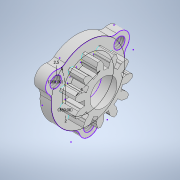
# Autodesk Inventor part: m1歯数11ギア6td6
Saved by Autodesk Inventor 2020.2 (Build 242310000, 310)
## iProperties
Created: 2020-02-29
Part Number: m1歯数11ギア6td6
Material: 一般
Document SubType Name: Modeling
Designer: aoyam
Density: 1 g/cm^3
Appearance: 既定
Author: aoyam
Autodesk Inventor part; units mm, degrees
ref_plane "YZ Plane" through (0, 0, 0) normal (1, 0, 0) x (0, 1, 0)
ref_plane "XZ Plane" through (0, 0, 0) normal (0, 1, 0) x (-1, 0, 0)
ref_plane "XY Plane" through (0, 0, 0) normal (0, 0, 1) x (1, 0, 0)
sketch "スケッチ1" plane through (0, 0, 0) normal (1, 0, 0) x (0, 1, 0)
  arc A0 (3.9405, 8.9701) -> (3.9064, 8.8492) centre (4.5356, 8.7369) ccw
  arc A1 (4.1405, 9.35) -> (3.9405, 8.9701) centre (5.6048, 8.3365) ccw
  arc A2 (4.786, 10.0383) -> (4.1405, 9.35) centre (6.7489, 7.5504) ccw
  arc A3 (2.588, 8.8492) -> (2.5538, 8.9701) centre (1.9587, 8.7369) ccw
  arc A4 (2.5538, 8.9701) -> (2.3538, 9.35) centre (0.8895, 8.3365) ccw
  arc A5 (2.3538, 9.35) -> (1.7083, 10.0383) centre (-0.2546, 7.5504) ccw
  arc A6 (3.7892, 7.9384) -> (2.7051, 7.9384) centre (3.2472, 3.7231) ccw
  arc A7 (1.7083, 10.0383) -> (1.1275, 9.8677) centre (3.2472, 3.7231) ccw
  line L0 (3.7892, 7.9384) -> (3.9064, 8.8492)
  line L1 (2.7051, 7.9384) -> (2.588, 8.8492)
  arc A8 (-0.1729, 7.7623) -> (-0.5466, 7.9738) centre (-1.2304, 6.3295) ccw
  arc A9 (-0.5466, 7.9738) -> (-1.4617, 8.2038) centre (-1.768, 5.0496) ccw
  arc A10 (-1.4617, 8.2038) -> (-1.8581, 7.7463) centre (3.2472, 3.7231) ccw
  arc A11 (0.9937, 8.512) -> (1.0303, 8.3918) centre (1.6204, 8.6376) ccw
  arc A12 (-0.0788, 7.679) -> (-0.1729, 7.7623) centre (-0.5474, 7.2444) ccw
  line L2 (0.5122, 6.9761) -> (-0.0788, 7.679)
  arc A13 (1.4242, 7.5623) -> (0.5122, 6.9761) centre (3.2472, 3.7231) ccw
  line L3 (1.4242, 7.5623) -> (1.0303, 8.3918)
  arc A14 (0.9565, 8.9398) -> (0.9937, 8.512) centre (2.7363, 8.8787) ccw
  arc A15 (1.1275, 9.8677) -> (0.9565, 8.9398) centre (4.1238, 8.836) ccw
  arc A16 (-1.8137, 5.2721) -> (-2.2424, 5.248) centre (-1.9287, 3.495) ccw
  arc A17 (-2.2424, 5.248) -> (-3.1366, 4.9467) centre (-1.689, 2.1277) ccw
  arc A18 (-3.1366, 4.9467) -> (-3.2228, 4.3475) centre (3.2472, 3.7231) ccw
  arc A19 (-1.2377, 6.5334) -> (-1.1419, 6.4522) centre (-0.7783, 6.9779) ccw
  arc A20 (-1.6895, 5.2529) -> (-1.8137, 5.2721) centre (-1.8488, 4.6339) ccw
  line L4 (-0.8124, 4.9811) -> (-1.6895, 5.2529)
  arc A21 (-0.362, 5.9672) -> (-0.8124, 4.9811) centre (3.2472, 3.7231) ccw
  line L5 (-0.362, 5.9672) -> (-1.1419, 6.4522)
  arc A22 (-1.5002, 6.8732) -> (-1.2377, 6.5334) centre (0.0301, 7.7841) ccw
  arc A23 (-1.8581, 7.7463) -> (-1.5002, 6.8732) centre (1.2204, 8.4983) ccw
  arc A24 (-1.8478, 2.2901) -> (-2.1954, 2.038) centre (-0.9838, 0.7329) ccw
  arc A25 (-2.1954, 2.038) -> (-2.7848, 1.3011) centre (-0.0429, -0.2878) ccw
  arc A26 (-2.7848, 1.3011) -> (-2.5333, 0.7505) centre (3.2472, 3.7231) ccw
  arc A27 (-2.0452, 3.6626) -> (-1.9206, 3.646) centre (-1.899, 4.2848) ccw
  arc A28 (-1.7329, 2.3411) -> (-1.8478, 2.2901) centre (-1.5323, 1.7342) ccw
  line L6 (-0.8481, 2.5866) -> (-1.7329, 2.3411)
  arc A29 (-1.0024, 3.6597) -> (-0.8481, 2.5866) centre (3.2472, 3.7231) ccw
  line L7 (-1.0024, 3.6597) -> (-1.9206, 3.646)
  arc A30 (-2.4497, 3.8065) -> (-2.0452, 3.6626) centre (-1.6548, 5.4002) ccw
  arc A31 (-3.2228, 4.3475) -> (-2.4497, 3.8065) centre (-1.0396, 6.6445) ccw
  arc A32 (-0.2643, -0.237) -> (-0.4204, -0.637) centre (1.3045, -1.0799) ccw
  arc A33 (-0.4204, -0.637) -> (-0.5178, -1.5755) centre (2.6478, -1.4298) ccw
  arc A34 (-0.5178, -1.5755) -> (-0.0086, -1.9028) centre (3.2472, 3.7231) ccw
  arc A35 (-1.1723, 0.811) -> (-1.0586, 0.8644) centre (-1.3858, 1.4134) ccw
  arc A36 (-0.1952, -0.132) -> (-0.2643, -0.237) centre (0.3017, -0.534) ccw
  line L8 (0.4164, 0.553) -> (-0.1952, -0.132)
  arc A37 (-0.2935, 1.3723) -> (0.4164, 0.553) centre (3.2472, 3.7231) ccw
  line L9 (-0.2935, 1.3723) -> (-1.0586, 0.8644)
  arc A38 (-1.5905, 0.7133) -> (-1.1723, 0.811) centre (-1.7833, 2.4837) ccw
  arc A39 (-2.5333, 0.7505) -> (-1.5905, 0.7133) centre (-1.9385, 3.8632) ccw
  arc A40 (2.4341, -1.5068) -> (2.519, -1.9277) centre (4.2096, -1.3677) ccw
  arc A41 (2.519, -1.9277) -> (2.9445, -2.7699) centre (5.5288, -0.9358) ccw
  arc A42 (2.9445, -2.7699) -> (3.5498, -2.7699) centre (3.2472, 3.7231) ccw
  arc A43 (1.1036, -1.1161) -> (1.1705, -1.0097) centre (0.5984, -0.7247) ccw
  arc A44 (2.4355, -1.3811) -> (2.4341, -1.5068) centre (3.0708, -1.4507) ccw
  line L10 (2.5797, -0.4742) -> (2.4355, -1.3811)
  arc A45 (1.5395, -0.1688) -> (2.5797, -0.4742) centre (3.2472, 3.7231) ccw
  line L11 (1.5395, -0.1688) -> (1.1705, -1.0097)
  arc A46 (0.8047, -1.4243) -> (1.1036, -1.1161) centre (-0.3147, -0.0392) ccw
  arc A47 (-0.0086, -1.9028) -> (0.8047, -1.4243) centre (-1.1911, 1.0373) ccw
  arc A48 (5.3907, -1.1161) -> (5.6896, -1.4243) centre (6.809, -0.0392) ccw
  arc A49 (5.6896, -1.4243) -> (6.5029, -1.9028) centre (7.6854, 1.0373) ccw
  arc A50 (6.5029, -1.9028) -> (7.0121, -1.5755) centre (3.2472, 3.7231) ccw
  arc A51 (4.0602, -1.5068) -> (4.0588, -1.3811) centre (3.4235, -1.4507) ccw
  arc A52 (5.3238, -1.0097) -> (5.3907, -1.1161) centre (5.896, -0.7247) ccw
  line L12 (4.9549, -0.1688) -> (5.3238, -1.0097)
  arc A53 (3.9146, -0.4742) -> (4.9549, -0.1688) centre (3.2472, 3.7231) ccw
  line L13 (3.9146, -0.4742) -> (4.0588, -1.3811)
  arc A54 (3.9753, -1.9277) -> (4.0602, -1.5068) centre (2.2848, -1.3677) ccw
  arc A55 (3.5498, -2.7699) -> (3.9753, -1.9277) centre (0.9655, -0.9358) ccw
  arc A56 (7.6666, 0.811) -> (8.0848, 0.7133) centre (8.2777, 2.4837) ccw
  arc A57 (8.0848, 0.7133) -> (9.0276, 0.7505) centre (8.4329, 3.8632) ccw
  arc A58 (9.0276, 0.7505) -> (9.2791, 1.3011) centre (3.2472, 3.7231) ccw
  arc A59 (6.7586, -0.237) -> (6.6895, -0.132) centre (6.1926, -0.534) ccw
  arc A60 (7.5529, 0.8644) -> (7.6666, 0.811) centre (7.8801, 1.4134) ccw
  line L14 (6.7878, 1.3723) -> (7.5529, 0.8644)
  arc A61 (6.0779, 0.553) -> (6.7878, 1.3723) centre (3.2472, 3.7231) ccw
  line L15 (6.0779, 0.553) -> (6.6895, -0.132)
  arc A62 (6.9147, -0.637) -> (6.7586, -0.237) centre (5.1898, -1.0799) ccw
  arc A63 (7.0121, -1.5755) -> (6.9147, -0.637) centre (3.8465, -1.4298) ccw
  arc A64 (8.5395, 3.6626) -> (8.944, 3.8065) centre (8.1491, 5.4002) ccw
  arc A65 (8.944, 3.8065) -> (9.7171, 4.3475) centre (7.5339, 6.6445) ccw
  arc A66 (9.7171, 4.3475) -> (9.6309, 4.9467) centre (3.2472, 3.7231) ccw
  arc A67 (8.3421, 2.2901) -> (8.2273, 2.3411) centre (8.0266, 1.7342) ccw
  arc A68 (8.4149, 3.646) -> (8.5395, 3.6626) centre (8.3933, 4.2848) ccw
  line L16 (7.4967, 3.6597) -> (8.4149, 3.646)
  arc A69 (7.3424, 2.5866) -> (7.4967, 3.6597) centre (3.2472, 3.7231) ccw
  line L17 (7.3424, 2.5866) -> (8.2273, 2.3411)
  arc A70 (8.6897, 2.038) -> (8.3421, 2.2901) centre (7.4781, 0.7329) ccw
  arc A71 (9.2791, 1.3011) -> (8.6897, 2.038) centre (6.5372, -0.2878) ccw
  arc A72 (7.732, 6.5334) -> (7.9945, 6.8732) centre (6.4643, 7.7841) ccw
  arc A73 (7.9945, 6.8732) -> (8.3524, 7.7463) centre (5.2739, 8.4983) ccw
  arc A74 (8.3524, 7.7463) -> (7.956, 8.2038) centre (3.2472, 3.7231) ccw
  arc A75 (8.3081, 5.2721) -> (8.1839, 5.2529) centre (8.3431, 4.6339) ccw
  arc A76 (7.6362, 6.4522) -> (7.732, 6.5334) centre (7.2727, 6.9779) ccw
  line L18 (6.8563, 5.9672) -> (7.6362, 6.4522)
  arc A77 (7.3067, 4.9811) -> (6.8563, 5.9672) centre (3.2472, 3.7231) ccw
  line L19 (7.3067, 4.9811) -> (8.1839, 5.2529)
  arc A78 (8.7367, 5.248) -> (8.3081, 5.2721) centre (8.4231, 3.495) ccw
  arc A79 (9.6309, 4.9467) -> (8.7367, 5.248) centre (8.1833, 2.1277) ccw
  arc A80 (5.5007, 8.512) -> (5.5378, 8.9398) centre (3.758, 8.8787) ccw
  arc A81 (5.5378, 8.9398) -> (5.3668, 9.8677) centre (2.3705, 8.836) ccw
  arc A82 (5.3668, 9.8677) -> (4.786, 10.0383) centre (3.2472, 3.7231) ccw
  arc A83 (6.6672, 7.7623) -> (6.5731, 7.679) centre (7.0417, 7.2444) ccw
  arc A84 (5.464, 8.3918) -> (5.5007, 8.512) centre (4.8739, 8.6376) ccw
  line L20 (5.0701, 7.5623) -> (5.464, 8.3918)
  arc A85 (5.9821, 6.9761) -> (5.0701, 7.5623) centre (3.2472, 3.7231) ccw
  line L21 (5.9821, 6.9761) -> (6.5731, 7.679)
  arc A86 (7.0409, 7.9738) -> (6.6672, 7.7623) centre (7.7247, 6.3295) ccw
  arc A87 (7.956, 8.2038) -> (7.0409, 7.9738) centre (8.2623, 5.0496) ccw
  circle A88 centre (3.2472, 3.7231) radius 3
  circle A89 centre (7.1594, 10.9864) radius 1.25
  arc A90 (9.3549, 10.4941) -> (5.5402, 12.5487) centre (7.1594, 10.9864) ccw
  arc A91 (9.3549, 10.4941) -> (9.7339, 8.8206) centre (11.3064, 10.0564) ccw
  arc A92 (3.9344, 11.9444) -> (5.5402, 12.5487) centre (4.101, 13.9374) ccw
  circle A93 centre (-4.9992, 3.4795) radius 1.25
  arc A94 (-5.6706, 5.627) -> (-4.4108, 6.792) centre (-6.2673, 7.5359) ccw
  arc A95 (-5.6706, 5.627) -> (-5.5426, 1.2961) centre (-4.9992, 3.4795) ccw
  arc A96 (-4.2163, 0.2076) -> (-5.5426, 1.2961) centre (-6.0257, -0.6447) ccw
  circle A97 centre (7.5813, -3.2967) radius 1.25
  arc A98 (6.0571, -4.9519) -> (4.4184, -4.4434) centre (4.7023, -6.4231) ccw
  arc A99 (6.0571, -4.9519) -> (9.7439, -2.6756) centre (7.5813, -3.2967) ccw
  arc A100 (10.0234, -0.9827) -> (9.7439, -2.6756) centre (11.6662, -2.1236) ccw
  arc A101 (10.0234, -0.9827) -> (9.7339, 8.8206) centre (3.2472, 3.7231) ccw
  arc A102 (3.9344, 11.9444) -> (-4.4108, 6.792) centre (3.2472, 3.7231) ccw
  arc A103 (-4.2163, 0.2076) -> (4.4184, -4.4434) centre (3.2472, 3.7231) ccw
  point P0 (0, 0)
  point P1 (5.4986, 8.5025)
  point P2 (5.538, 8.9335)
  point P3 (5.3668, 9.8677)
  point P4 (4.786, 10.0383)
  point P5 (4.137, 9.3449)
  point P6 (3.937, 8.9611)
  point P7 (3.9064, 8.8492)
  point P8 (3.7892, 7.9384)
  point P9 (2.7051, 7.9384)
  point P10 (2.5573, 8.9611)
  point P11 (2.3573, 9.3449)
  point P12 (1.7083, 10.0383)
  point P13 (1.1275, 9.8677)
  point P14 (0.9563, 8.9335)
  point P15 (0.9956, 8.5025)
  point P16 (1.4242, 7.5623)
  point P17 (0.5122, 6.9761)
  point P18 (-0.1651, 7.7565)
  point P19 (-0.5408, 7.9714)
  point P20 (-1.4617, 8.2038)
  point P21 (-1.8581, 7.7463)
  point P22 (-1.497, 6.8679)
  point P23 (-1.2309, 6.5265)
  point P24 (-1.1419, 6.4522)
  point P25 (-0.362, 5.9672)
  point P26 (-0.8124, 4.9811)
  point P27 (-1.8041, 5.2714)
  point P28 (-2.2363, 5.2491)
  point P29 (-3.1366, 4.9467)
  point P30 (-3.2228, 4.3475)
  point P31 (-2.4441, 3.8038)
  point P32 (-2.0357, 3.6605)
  point P33 (-1.9206, 3.646)
  point P34 (-1.0024, 3.6597)
  point P35 (-0.8481, 2.5866)
  point P36 (-1.8393, 2.2947)
  point P37 (-2.1908, 2.0422)
  point P38 (-2.7848, 1.3011)
  point P39 (-2.5333, 0.7505)
  point P40 (-1.5842, 0.714)
  point P41 (-1.1632, 0.8143)
  point P42 (-0.2597, -0.2285)
  point P43 (-0.4188, -0.6309)
  point P44 (-0.5178, -1.5755)
  point P45 (-0.0086, -1.9028)
  point P46 (0.8095, -1.4203)
  point P47 (1.1095, -1.1084)
  point P48 (2.5797, -0.4742)
  point P49 (2.4334, -1.4971)
  point P50 (2.5171, -1.9217)
  point P51 (2.9445, -2.7699)
  point P52 (3.5498, -2.7699)
  point P53 (3.9772, -1.9217)
  point P54 (4.061, -1.4971)
  point P55 (5.3848, -1.1084)
  point P56 (5.6848, -1.4203)
  point P57 (6.5029, -1.9028)
  point P58 (7.0121, -1.5755)
  point P59 (6.9131, -0.6309)
  point P60 (6.754, -0.2285)
  point P61 (6.6895, -0.132)
  point P62 (6.0779, 0.553)
  point P63 (6.7878, 1.3723)
  point P64 (7.6576, 0.8143)
  point P65 (8.0786, 0.714)
  point P66 (9.0276, 0.7505)
  point P67 (9.2791, 1.3011)
  point P68 (8.6851, 2.0422)
  point P69 (8.3337, 2.2948)
  point P70 (8.2273, 2.3411)
  point P71 (8.53, 3.6605)
  point P72 (8.9384, 3.8038)
  point P73 (9.7171, 4.3475)
  point P74 (9.6309, 4.9467)
  point P75 (8.7306, 5.2491)
  point P76 (8.2984, 5.2715)
  point P77 (8.1839, 5.2529)
  point P78 (7.3067, 4.9811)
  point P79 (7.7252, 6.5266)
  point P80 (7.9913, 6.8679)
  point P81 (8.3524, 7.7463)
  point P82 (7.956, 8.2038)
  point P83 (7.0351, 7.9714)
  point P84 (6.6594, 7.7566)
  point P85 (-0.2643, -0.237)
  point P86 (-0.4204, -0.637)
  point P87 (0.8047, -1.4243)
  point P88 (1.1095, -1.1084)
  point P89 (2.4334, -1.4971)
  point P90 (2.519, -1.9277)
  point P91 (3.9753, -1.9277)
  point P92 (4.0602, -1.5068)
  point P93 (5.3848, -1.1084)
  point P94 (5.6896, -1.4243)
  point P95 (6.9147, -0.637)
  point P96 (6.7586, -0.237)
  point P97 (7.6666, 0.811)
  point P98 (8.0848, 0.7133)
  point P99 (8.6851, 2.0422)
  point P100 (8.3337, 2.2948)
  point P101 (8.5395, 3.6626)
  point P102 (8.944, 3.8065)
  point P103 (8.7306, 5.2491)
  point P104 (8.3081, 5.2721)
  point P105 (7.732, 6.5334)
  point P106 (7.9945, 6.8732)
  point P107 (7.0409, 7.9738)
  point P108 (6.6672, 7.7623)
  point P109 (5.5007, 8.512)
  point P110 (5.538, 8.9335)
  point P111 (4.1405, 9.35)
  point P112 (3.9405, 8.9701)
  point P113 (2.5573, 8.9611)
  point P114 (2.3538, 9.35)
  point P115 (0.9565, 8.9398)
  point P116 (0.9937, 8.512)
  point P117 (-0.1729, 7.7623)
  point P118 (-0.5466, 7.9738)
  point P119 (-1.5002, 6.8732)
  point P120 (-1.2309, 6.5265)
  point P121 (-1.8041, 5.2714)
  point P122 (-2.2424, 5.248)
  point P123 (-2.4441, 3.8038)
  point P124 (-2.0357, 3.6605)
  point P125 (-1.8478, 2.2901)
  point P126 (-2.1908, 2.0422)
  point P127 (-1.5905, 0.7133)
  point P128 (-1.1723, 0.811)
  dimension "d2" = 360
  dimension "d6" = 6
  dimension "d8" = 2.5
  dimension "d10" = 2
  dimension "d13" = 360
  constraints: 200 point on circle, 104 centre point, 44 end point, 4 coincident, 2 tangent, 1 equal radius, 451 other
  measures "d6" diameter of A88
  measures "d8" diameter of A89
  measures "d10" radius of A91
extrude "押し出し1" add sketch "スケッチ1" along normal blind 3.5 contours A1 A2 A82 A81 A80 A84 L20 A85 L21 A83 A86 A87 A74 A73 A72 A76 L18 A77 L19 A75 A78 A79 A66 A65 A64 A68 L16 A69 L17 A67 A70 A71 A58 A57 A56 A60 L14 A61 L15 A59 A62 A63 A50 A49 A48 A52 L12 A53 L13 A51 A54 A55 A42 A41 A40 A44 L10 A45 L11 A43 A46 A47 A34 A33 A32 A36 L8 A37 L9 A35 A38 A39 A26 A25 A24 A28 L6 A29 L7 A27 A30 A31 A18 A17 A16 A20 L4 A21 L5 A19 A22 A23 A10 A9 A8 A12 L2 A13 L3 A11 A14 A15 A7 A5 A4 A3 L1 A6 L0 A0
extrude "押し出し2" add sketch "スケッチ1" against normal blind 2.5 contours A1 A2 A82 A81 A80 A84 L20 A85 L21 A83 A86 A87 A74 A73 A72 A76 L18 A77 L19 A75 A78 A79 A66 A65 A64 A68 L16 A69 L17 A67 A70 A71 A58 A57 A56 A60 L14 A61 L15 A59 A62 A63 A50 A49 A48 A52 L12 A53 L13 A51 A54 A55 A42 A41 A40 A44 L10 A45 L11 A43 A46 A47 A34 A33 A32 A36 L8 A37 L9 A35 A38 A39 A26 A25 A24 A28 L6 A29 L7 A27 A30 A31 A18 A17 A16 A20 L4 A21 L5 A19 A22 A23 A10 A9 A8 A12 L2 A13 L3 A11 A14 A15 A7 A5 A4 A3 L1 A6 L0 A0 | A91 A101 A100 A99 A98 A103 A96 A95 A94 A102 A92 A90
thread "ねじ1" size "M3x0.5" class "6H" standard "ANSI Metric M Profile" full length
thread "ねじ2" size "M3x0.5" class "6H" standard "ANSI Metric M Profile" full length
thread "ねじ3" size "M3x0.5" class "6H" standard "ANSI Metric M Profile" full length
